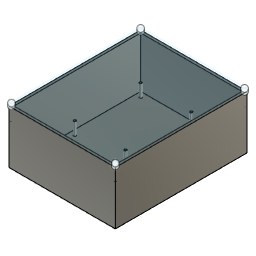
Screw Box v2 (Autodesk Fusion 360 design; units mm, degrees)
Autodesk Fusion 360 part; units mm, degrees
sketch "Sketch1" plane through (0, 0, 0) normal (0, 0, 1) x (1, 0, 0)
  line L0 (0, 0) -> (101.6, 0)
  line L1 (101.6, 0) -> (101.6, 127)
  line L2 (101.6, 127) -> (0, 127)
  line L3 (0, 127) -> (0, 0)
  circle A0 centre (2.54, 2.54) radius 0.762
  circle A1 centre (48.26, 2.54) radius 0.762
  circle A2 centre (2.54, 73.66) radius 0.762
  circle A3 centre (48.26, 73.66) radius 0.762
  circle A4 centre (2.54, 73.66) radius 1.27
  circle A5 centre (48.26, 73.66) radius 1.27
  circle A6 centre (2.54, 2.54) radius 1.27
  dimension "d1" = 101.6
  dimension "d2" = 127
  dimension "d3" = 1.524
  dimension "d4" = 1.524
  dimension "d5" = 1.524
  dimension "d6" = 1.524
  dimension "d7" = 2.54
  dimension "d8" = 2.54
  dimension "d9" = 2.54
  constraint horizontal L0
  constraint vertical L1
  constraint horizontal L2
  constraint vertical L3
  constraint coincident L0.start L3.end
  constraint concentric A2 A4
  constraint concentric A3 A5
  constraint concentric A0 A6
  measures "d1" distance of L0.start L0.end
  measures "d2" distance of L0.start L2.end
  measures "d3" diameter of A0
  measures "d4" diameter of A1
  measures "d5" diameter of A2
  measures "d6" diameter of A3
  measures "d7" diameter of A4
  measures "d8" diameter of A5
  measures "d9" diameter of A6
extrude "Extrude1" add sketch "Sketch1" along normal blind 2.54 contours L0 L1 L2 L3 | A0 | A1 | A2 | A3 | A4 | A5 | A6 makes body 1
move_body "Move1" bodies 1 to x (1, 0, 0) y (0, 1, 0) z (0, 0, 1) at (0, -63.5, 0)
move_body "Move2" bodies 1 to x (1, 0, 0) y (0, 1, 0) z (0, 0, 1) at (0, -63.5, 0)
sketch "Sketch2" plane through (0, 0, 2.54) normal (0, 0, 1) x (-1, 0, 0)
  line L0 (0, 0) -> (0, 127)
  line L1 (0, 127) -> (-101.6, 127)
  line L2 (-101.6, 127) -> (-101.6, 0)
  line L3 (-101.6, 0) -> (0, 0)
  circle A0 centre (-2.54, 2.54) radius 0.762
  circle A1 centre (-2.54, 73.66) radius 0.762
  circle A2 centre (-48.26, 2.54) radius 0.762
  circle A3 centre (-48.26, 73.66) radius 0.762
  circle A4 centre (-48.26, 73.66) radius 1.27
  circle A5 centre (-2.54, 73.66) radius 1.27
  circle A6 centre (-48.26, 2.54) radius 1.27
  circle A7 centre (-2.54, 2.54) radius 1.27
  dimension "d12" = 1.524
  dimension "d13" = 1.524
  dimension "d14" = 1.524
  dimension "d15" = 1.524
  dimension "d16" = 2.54
  dimension "d17" = 2.54
  dimension "d18" = 2.54
  dimension "d19" = 2.54
  constraint concentric A3 A4
  constraint concentric A1 A5
  constraint concentric A2 A6
  constraint concentric A0 A7
  measures "d12" diameter of A0
  measures "d13" diameter of A1
  measures "d14" diameter of A2
  measures "d15" diameter of A3
  measures "d16" diameter of A4
  measures "d17" diameter of A5
  measures "d18" diameter of A6
  measures "d19" diameter of A7
extrude "Extrude2" add sketch "Sketch2" along normal blind 6.35 contours A4 | A5 | A6 | A7 bodies 1
sketch "Sketch3" plane through (0, 0, 2.54) normal (0, 0, 1) x (-1, 0, 0)
  circle A0 centre (-2.54, 73.66) radius 1.27
  circle A1 centre (-48.26, 73.66) radius 1.27
  line L0 (0, 0) -> (0, 127)
  line L1 (0, 127) -> (-101.6, 127)
  line L2 (-101.6, 127) -> (-101.6, 0)
  line L3 (-101.6, 0) -> (0, 0)
  circle A2 centre (-2.54, 2.54) radius 1.27
  circle A3 centre (-48.26, 2.54) radius 1.27
  line L4 (2.54, -2.54) -> (-104.14, -2.54)
  line L5 (-104.14, -2.54) -> (-104.14, 129.54)
  line L6 (-104.14, 129.54) -> (2.54, 129.54)
  line L7 (2.54, 129.54) -> (2.54, -2.54)
  line L8 (-101.6, 127) -> (0, 127)
  line L9 (0, 127) -> (0, 0)
  line L10 (0, 0) -> (-101.6, 0)
  line L11 (-101.6, 0) -> (-101.6, 127)
  constraint horizontal L4
  constraint vertical L5
  constraint horizontal L6
  constraint vertical L7
  constraint horizontal L8
  constraint vertical L9
  constraint horizontal L10
  constraint vertical L11
  constraint coincident L0.start L3.end
  constraint coincident L1.end L2.start
extrude "Extrude3" add sketch "Sketch3" along normal blind 50.8 separate body contours L4 L5 L6 L7 makes body 2
extrude "Extrude4" add 1 faces at (103.2933, -84.6667, 2.54) along direction (0, 0, -1) blind 2.54 on bodies 2 bodies 2 1
sketch "Sketch4" plane through (0, 0, 0) normal (1, 0, 0) x (0, 1, 0)
sketch "Sketch5" plane through (0, 0, 0) normal (1, 0, 0) x (0, 1, 0)
  line L0 (-127, 2.54) -> (0, 2.54)
  line L1 (0, 2.54) -> (0, 53.34)
  line L2 (0, 53.34) -> (-127, 53.34)
  line L3 (-127, 53.34) -> (-127, 2.54)
delete_face "DeleteFace1" 1 faces at (46.9963, -73.5336, 6.7733) on bodies 2
delete_face "DeleteFace2" 1 faces at (1.2763, -73.5336, 6.7733) on bodies 2
delete_face "DeleteFace3" 1 faces at (46.9916, -2.4767, 4.6567) on bodies 2
delete_face "DeleteFace4" 1 faces at (1.2763, -2.4135, 6.7733) on bodies 2
sketch "Sketch6" plane through (0, 0, 2.54) normal (0, 0, 1) x (-1, 0, 0)
  line L0 (0, 0) -> (0, 127)
  line L1 (0, 127) -> (-101.6, 127)
  line L2 (-101.6, 127) -> (-101.6, 0)
  line L3 (-101.6, 0) -> (0, 0)
  circle A0 centre (-5.08, 5.08) radius 1.27
  circle A1 centre (-55.88, 5.08) radius 1.27
  circle A2 centre (-5.08, 71.12) radius 1.27
  circle A3 centre (-55.88, 71.12) radius 1.27
  dimension "d26" = 2.54
  dimension "d27" = 2.54
  dimension "d28" = 2.54
  dimension "d29" = 2.54
  measures "d26" diameter of A0
  measures "d27" diameter of A1
  measures "d28" diameter of A2
  measures "d29" diameter of A3
extrude "Extrude5" add sketch "Sketch6" along normal blind 12.7 contours A0 | A1 | A2 | A3 bodies 2
hole "Hole1" at (55.88, -5.08, 15.24) direction (0, 0, -1) diameter 1.6256 depth 12.7 tip angle 180 bodies 2
thread "Thread1" "ISO Metric profile 2.0 M2x0.4 6H"
hole "Hole2" at (5.08, -5.08, 15.24) direction (0, 0, -1) diameter 1.6256 depth 12.7 tip angle 180 bodies 2
thread "Thread2" "ISO Metric profile 2.0 M2x0.4 6H"
hole "Hole3" at (55.88, -71.12, 15.24) direction (0, 0, -1) diameter 1.6256 depth 12.7 tip angle 180 bodies 2
thread "Thread3" "ISO Metric profile 2.0 M2x0.4 6H"
hole "Hole4" at (5.08, -71.12, 15.24) direction (0, 0, -1) diameter 1.6256 depth 12.7 tip angle 180 bodies 2
thread "Thread4" "ISO Metric profile 2.0 M2x0.4 6H"
sketch "Sketch7" plane through (0, 0, 0) normal (0, 0, 1) x (1, 0, 0)
  line L0 (-2.54, 2.54) -> (104.14, 2.54)
  line L1 (104.14, 2.54) -> (104.14, -129.54)
  line L2 (104.14, -129.54) -> (-2.54, -129.54)
  line L3 (-2.54, -129.54) -> (-2.54, 2.54)
  constraint horizontal L0
  constraint vertical L1
  constraint horizontal L2
  constraint vertical L3
extrude "Extrude6" add sketch "Sketch7" along normal blind 2.54 separate body makes body 3
move_body "Move3" bodies 3 to x (1, 0, 0) y (0, 1, 0) z (0, 0, 1) at (0, 0, 53.34)
sketch "Sketch8" plane through (0, 0, 53.34) normal (0, 0, 1) x (-1, 0, 0)
  line L0 (0, 0) -> (-101.6, 0)
  line L1 (-101.6, 0) -> (-101.6, 127)
  line L2 (-101.6, 127) -> (0, 127)
  line L3 (0, 127) -> (0, 0)
  line L4 (2.54, 129.54) -> (-104.14, 129.54)
  line L5 (-104.14, 129.54) -> (-104.14, -2.54)
  line L6 (-104.14, -2.54) -> (2.54, -2.54)
  line L7 (2.54, -2.54) -> (2.54, 129.54)
  circle A0 centre (-102.87, -1.27) radius 1.0222
  circle A1 centre (-102.87, 128.27) radius 1.016
  circle A2 centre (1.27, 128.27) radius 1.016
  circle A3 centre (1.27, -1.27) radius 1.0163
  dimension "d46" = 2.032
  measures "d46" diameter of A2
hole "Hole5" at (102.87, -128.27, 53.34) direction (0, 0, -1) diameter 1.6256 depth 12.7 tip angle 180 bodies 2
thread "Thread5" "ISO Metric profile 2.0 M2x0.4 6H"
hole "Hole6" at (-1.27, -128.27, 53.34) direction (0, 0, -1) diameter 1.6256 depth 12.7 tip angle 180 bodies 2
thread "Thread6" "ISO Metric profile 2.0 M2x0.4 6H"
hole "Hole7" at (-1.27, 1.27, 53.34) direction (0, 0, -1) diameter 1.6256 depth 12.7 tip angle 180 bodies 2
thread "Thread7" "ISO Metric profile 2.0 M2x0.4 6H"
hole "Hole8" at (102.87, 1.27, 53.34) direction (0, 0, -1) diameter 1.6256 depth 12.7 tip angle 180 bodies 2
thread "Thread8" "ISO Metric profile 2.0 M2x0.4 6H"
sketch "Sketch9" plane through (0, 0, 55.88) normal (0, 0, 1) x (-1, 0, 0)
  line L0 (2.54, 129.54) -> (-104.14, 129.54)
  line L1 (-104.14, 129.54) -> (-104.14, -2.54)
  line L2 (-104.14, -2.54) -> (2.54, -2.54)
  line L3 (2.54, -2.54) -> (2.54, 129.54)
  circle A0 centre (-102.87, -1.27) radius 1.016
  circle A1 centre (-102.87, 128.27) radius 1.016
  circle A2 centre (1.27, 128.27) radius 1.016
  circle A3 centre (1.27, -1.27) radius 1.016
hole "Hole9" at (-1.27, 1.27, 55.88) direction (0, 0, -1) diameter 1.6256 depth 55.88 tip angle 180 counterbore diameter 4.4 counterbore depth 2 bodies 2 3
thread "Thread9" "ISO Metric profile 2.0 M2x0.4 6H"
hole "Hole10" at (-1.2295, -128.2703, 55.88) direction (0, 0, -1) diameter 1.6256 depth 2.54 tip angle 180 counterbore diameter 4.3942 counterbore depth 2.0066 bodies 3
thread "Thread10" "ISO Metric profile 2.0 M2x0.4 6H"
hole "Hole11" at (102.8982, -128.2699, 55.88) direction (0, 0, -1) diameter 1.6256 depth 2.54 tip angle 180 counterbore diameter 4.3942 counterbore depth 2.0066 bodies 3
thread "Thread11" "ISO Metric profile 2.0 M2x0.4 6H"
hole "Hole12" at (102.87, 1.27, 55.88) direction (0, 0, -1) diameter 1.6256 depth 2.54 tip angle 180 counterbore diameter 4.3942 counterbore depth 2.0066 bodies 3
thread "Thread12" "ISO Metric profile 2.0 M2x0.4 6H"
hidden bodies 3
